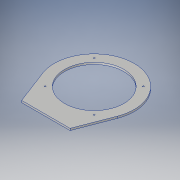
# Autodesk Inventor part: Turret Base Plate
Saved by Autodesk Inventor 2019.4 (Build 234330000, 330)
## iProperties
Created: 2020-01-06
Part Number: Turret Base Plate
Material: Aluminum 6061
Document SubType Name: Modeling
Designer: admin
Density: 2.7 g/cm^3
Appearance: Aluminum - Flat
Author: admin
Autodesk Inventor part; units mm, degrees
ref_plane "YZ Plane" through (0, 0, 0) normal (1, 0, 0) x (0, 1, 0)
ref_plane "XZ Plane" through (0, 0, 0) normal (0, 1, 0) x (-1, 0, 0)
ref_plane "XY Plane" through (0, 0, 0) normal (0, 0, 1) x (1, 0, 0)
sketch "Sketch1" plane through (0, 0, 0) normal (0, 1, 0) x (-1, 0, 0)
  circle A0 centre (0, 0) radius 122.5
  arc A1 (154.0532, 59.0984) -> (-154.0532, 59.0984) centre (0, 0) ccw construction
  line L0 (-154.0532, 59.0984) -> (-100, 200)
  line L1 (-100, 200) -> (100, 200)
  line L2 (100, 200) -> (154.0532, 59.0984)
  line L3 (0, 200) -> (0, 0) construction
  arc A2 (-154.0532, 59.0984) -> (154.0532, 59.0984) centre (0, 0) ccw
  line L4 (-101.5, 101.5) -> (101.5, 101.5) construction
  line L5 (101.5, 101.5) -> (101.5, -101.5) construction
  line L6 (101.5, -101.5) -> (-101.5, -101.5) construction
  line L7 (-101.5, -101.5) -> (-101.5, 101.5) construction
  line L8 (-101.5, 101.5) -> (101.5, -101.5) construction
  line L9 (101.5, 101.5) -> (-101.5, -101.5) construction
  circle A3 centre (101.5, -101.5) radius 2.75
  circle A4 centre (-101.5, -101.5) radius 2.75
  circle A5 centre (-101.5, 101.5) radius 2.75
  circle A6 centre (101.5, 101.5) radius 2.75
  dimension "d0" = 245
  dimension "d1" = 330
  dimension "d2" = 200
  dimension "d3" = 200
  dimension "d6" = 203
  dimension "d7" = 5.5
  dimension "d8" = 5.5
  dimension "d9" = 5.5
  dimension "d10" = 5.5
  constraints: 20 end point, 7 centre point, 6 coincident, 4 point on circle, 3 midpoint, 3 perpendicular, 2 horizontal, 2 parallel, 2 tangent
  measures "d0" diameter of A0
  measures "d1" diameter of A1
  measures "d2" distance from line of L1 point (0, 0)
  measures "d3" distance of L0.end L1.end
  measures "d6" distance of L4.end L5.end
  measures "d7" diameter of A3
  measures "d8" diameter of A4
  measures "d9" diameter of A5
  measures "d10" diameter of A6
extrude "Extrusion1" add sketch "Sketch1" along normal blind 8
body "Solid1"
